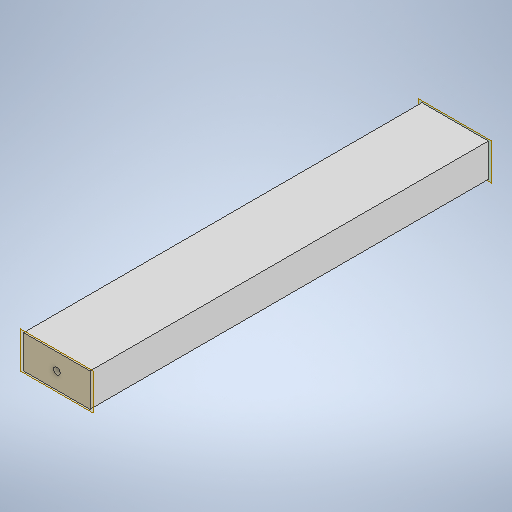
# Autodesk Inventor part: block1
Saved by Autodesk Inventor 2025.1 (Build 291241000, 241)
## iProperties
Created: 2024-11-25
Part Number: block1
Material: 一般
Document SubType Name: Modeling
Designer: dell
Density: 1 g/cm^3
Appearance: 既定
Author: dell
Autodesk Inventor part; units mm, degrees
ref_plane "YZ Plane" through (0, 0, 0) normal (1, 0, 0) x (0, 1, 0)
ref_plane "XZ Plane" through (0, 0, 0) normal (0, 1, 0) x (-1, 0, 0)
ref_plane "XY Plane" through (0, 0, 0) normal (0, 0, 1) x (1, 0, 0)
sketch "スケッチ1" plane through (0, 0, 0) normal (0, 1, 0) x (-1, 0, 0)
  line L0 (0, 0) -> (-50, 0)
  line L1 (-50, 0) -> (-50, -300)
  line L2 (-50, -300) -> (0, -300)
  line L3 (0, -300) -> (0, 0)
  dimension "d0" = 50
  dimension "d1" = 300
  constraints: 8 end point, 2 parallel, 1 horizontal, 1 perpendicular
  measures "d0" distance of L2.end L1.end
  measures "d1" distance of L1.end L0.end
extrude "押し出し1" add sketch "スケッチ1" along normal blind 25
ref_plane "作業平面1" through (0, 0, 0) normal (0, 0, 1) x (1, 0, 0)
sketch "スケッチ2" plane through (0, 0, 0) normal (0, 0, 1) x (1, 0, 0)
  point P0 (0, 0)
  point P1 (25, 12.5)
ref_plane "作業平面2" through (50, 0, -300) normal (0, 0, -1) x (-1, 0, 0)
sketch "スケッチ3" plane through (50, 0, -300) normal (0, 0, -1) x (-1, 0, 0)
  point P0 (50, 0)
  point P1 (25, 12.5)
hole "穴1" at (25, 12.5, -300) direction (0, 0, 1) diameter 5.1 depth 10
hole "穴2" at (25, 12.5, 0) direction (0, 0, -1) diameter 5.1 depth 10
